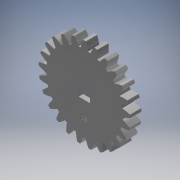
# Autodesk Inventor part: 25_teeth
Saved by Autodesk Inventor 2019 (Build 230136000, 136)
## iProperties
Created: 2020-02-24
Part Number: 25_teeth
Material: Steel
Document SubType Name: Modeling
Designer: Jeff
Categories: <?xml version="1.0" encoding="UTF-16"?> <MemberInstance><Categories><FamilyTemplate><FamilyTemplateParameter ValueType="xs:double" Id="1" ObjectReferenceKey="da_z" ObjectType="kUserParameterObject"/><FamilyTemplateParameter ValueType="xs:double" Id="2" ObjectReferenceKey="da_b" ObjectType="kUserParameterObject"/><FamilyTemplateParameter ValueType="xs:double" Id="3" ObjectReferenceKey="da_beta" ObjectType="kUserParameterObject"/><FamilyTemplateParameter ValueType="xs:double" Id="4" ObjectReferenceKey="da_da" ObjectType="kUserParameterObject"/><FamilyTemplateParameter ValueType="xs:double" Id="5" ObjectReferenceKey="da_aw" ObjectType="kUserParameterObject"/><FamilyTemplateParameter ValueType="xs:string" Id="6" ObjectReferenceKey="EAIAABAAAACIAQAAAAAAAIAAAAAAAAAA" ObjectType="83910656" SubObjectId="SurfaceGeometry"/></FamilyTemplate><ParamToTemplateMap><ParamToTemplate CategoryParameter="//CategoryParameter[@InternalName='046C89C9-8512-4d59-83FE-43B91F4F132A']" TemplateParameter="1"/><ParamToTemplate CategoryParameter="//CategoryParameter[@InternalName='2552DF32-E462-4b46-AEBF-C6C7768E72AC']" TemplateParameter="2"/><ParamToTemplate CategoryParameter="//CategoryParameter[@InternalName='C9EE641D-15FC-4fae-A226-E94C4372FDD7']" TemplateParameter="3"/><ParamToTemplate><ParamToTemplate CategoryParameter="//CategoryParameter[@InternalName='00B6519A-459B-49c7-AD84-2E56D39A5744']" ConstantValue="0.000000"/></ParamToTemplate><ParamToTemplate><ParamToTemplate CategoryParameter="//CategoryParameter[@InternalName='04B31F0E-C7A6-4894-AA32-9629BEFACF47']" ConstantValue="1.000000"/></ParamToTemplate><ParamToTemplate><ParamToTemplate CategoryParameter="//CategoryParameter[@InternalName='43CBEC2E-7847-49e7-A936-2F7889FCB2D9']" ConstantValue="0.250000"/></ParamToTemplate><ParamToTemplate><ParamToTemplate CategoryParameter="//CategoryParameter[@InternalName='B1EFC894-105D-4ebd-86BF-FA20ED196853']" ConstantValue="0.350000"/></ParamToTemplate><ParamToTemplate><ParamToTemplate CategoryParameter="//CategoryParameter[@InternalName='51175063-3D10-4879-93E8-6246FE8B403D']" ConstantValue="2060000000.000000"/></ParamToTemplate><ParamToTemplate><ParamToTemplate CategoryParameter="//CategoryParameter[@InternalName='A3A52E27-4454-46a9-B0BD-C932399B70AF']" ConstantValue="0.300000"/></ParamToTemplate><ParamToTemplate><ParamToTemplate CategoryParameter="//CategoryParameter[@InternalName='91B76062-C214-41d9-B1B9-14D2AB99603D']" ConstantValue="0.300000"/></ParamToTemplate><ParamToTemplate><ParamToTemplate CategoryParameter="//CategoryParameter[@InternalName='374E806E-8B8A-4dda-A9AA-1039D6500AD2']" ConstantValue="3.333333"/></ParamToTemplate><ParamToTemplate><ParamToTemplate CategoryParameter="//CategoryParameter[@InternalName='2D373A89-B862-43d6-8D0B-0CBF12AB9F6C']" ConstantValue="0.349066"/></ParamToTemplate><ParamToTemplate CategoryParameter="//CategoryParameter[@InternalName='37777632-D6A2-4fac-9D53-DB8ACD95C989']" TemplateParameter="4"/><ParamToTemplate CategoryParameter="//CategoryParameter[@InternalName='FD1017F1-B727-4f7e-9707-0F86F1FF9423']" TemplateParameter="5"/><ParamToTemplate><ParamToTemplate CategoryParameter="//CategoryParameter[@InternalName='9E1B4470-B2D3-4ff1-B813-535BB4CDF51A']" ConstantValue="3520000.000000"/></ParamToTemplate><ParamToTemplate><ParamToTemplate CategoryParameter="//CategoryParameter[@InternalName='F8452263-BFF6-458c-9FB1-07C4B99E95CD']" ConstantValue="11400000.000000"/></ParamToTemplate><ParamToTemplate><ParamToTemplate CategoryParameter="//CategoryParameter[@InternalName='3E3BB259-FD49-497f-8171-6EBC954A3479']" ConstantValue="2.000000"/></ParamToTemplate><ParamToTemplate CategoryParameter="//CategoryParameter[@InternalName='27C3BAF2-7550-4e4b-AE2C-0DB134B7D9B7']" TemplateParameter="6"/></ParamToTemplateMap><Category DisplayName="Gear" InternalName="DC85795E-93AB-48d5-8EEE-5A27447B64BD" Mnemonic="Gear"><CategoryParameter DisplayName="z" InternalName="046C89C9-8512-4d59-83FE-43B91F4F132A" Mnemonic="z"/><CategoryParameter DisplayName="b" InternalName="2552DF32-E462-4b46-AEBF-C6C7768E72AC" Mnemonic="b"/><CategoryParameter DisplayName="||b|" InternalName="C9EE641D-15FC-4fae-A226-E94C4372FDD7" Mnemonic="beta"/><CategoryParameter DisplayName="x" InternalName="00B6519A-459B-49c7-AD84-2E56D39A5744" Mnemonic="x"/><CategoryParameter DisplayName="a*" InternalName="04B31F0E-C7A6-4894-AA32-9629BEFACF47" Mnemonic="a"/><CategoryParameter DisplayName="c*" InternalName="43CBEC2E-7847-49e7-A936-2F7889FCB2D9" Mnemonic="c"/><CategoryParameter DisplayName="r|.f|*" InternalName="B1EFC894-105D-4ebd-86BF-FA20ED196853" Mnemonic="rf"/><CategoryParameter DisplayName="E" InternalName="51175063-3D10-4879-93E8-6246FE8B403D" Mnemonic="E"/><CategoryParameter DisplayName="||m|" InternalName="A3A52E27-4454-46a9-B0BD-C932399B70AF" Mnemonic="mi"/><Category DisplayName="SpurGear" InternalName="26C5A22E-A91E-4dfd-A3B3-23CCAFAE1764" Mnemonic="SpurGear"><CategoryParameter DisplayName="m" InternalName="91B76062-C214-41d9-B1B9-14D2AB99603D" Mnemonic="m"/><CategoryParameter DisplayName="P" InternalName="374E806E-8B8A-4dda-A9AA-1039D6500AD2" Mnemonic="PP"/><CategoryParameter DisplayName="||a|" InternalName="2D373A89-B862-43d6-8D0B-0CBF12AB9F6C" Mnemonic="alpha"/><CategoryParameter DisplayName="d|.a|" InternalName="37777632-D6A2-4fac-9D53-DB8ACD95C989" Mnemonic="da"/><CategoryParameter DisplayName="a|.w|" InternalName="FD1017F1-B727-4f7e-9707-0F86F1FF9423" Mnemonic="aw"/><CategoryParameter DisplayName="||s||.Flim|" InternalName="9E1B4470-B2D3-4ff1-B813-535BB4CDF51A" Mnemonic="sFlim"/><CategoryParameter DisplayName="||s||.Hlim|" InternalName="F8452263-BFF6-458c-9FB1-07C4B99E95CD" Mnemonic="sHlim"/><CategoryParameter DisplayName="type" InternalName="3E3BB259-FD49-497f-8171-6EBC954A3479" Mnemonic="type"/><CategoryParameter DisplayName="PitchDiameter" InternalName="27C3BAF2-7550-4e4b-AE2C-0DB134B7D9B7" Mnemonic="IDS_PITCHDIAM"/></Category></Category></Categories></MemberInstance>
Density: 1 g/cm^3
Appearance: Steel
CustomPartVersion: 1
Author: Jeff
Autodesk Inventor part; units mm, degrees
sketch "Sketch1" plane through (0, 0, 0) normal (0, 0, 1) x (1, 0, 0)
  circle A0 centre (0, 0) radius 40.5
  dimension "d0" = 81
  constraints: 1 centre point
  measures "d0" diameter of A0
extrude "Extrusion1" add sketch "Sketch1" along normal blind 10
ref_plane "Work Plane2" through (0, 0, 5) normal (0, 0, 1) x (1, 0, 0)
sketch "Sketch2" plane through (0, 0, 0) normal (0, 0, -1) x (-1, 0, 0)
  circle A0 centre (0, 0) radius 40.5 projected
  circle A1 centre (0, 0) radius 37.5
  dimension "d3" = 75
  constraints: 1 centre point, 1 coincident
  measures "d3" diameter of A1
surface extrude "Pitch Diameter" sketch "Sketch2" against normal through all shown no curves A1
ref_plane "Work Plane8" through (0, 0, 0) normal (0.9921147, 0.1253332, 0) x (0, 0, 1)
ref_plane "Work Plane9" through (0, 0, 0) normal (1, 0, 0) x (0, 1, 0)
spur gear teeth "Spur Gear" teeth 25 pitch diameter 75 tip diameter 81 root diameter 67.5 face width 10 start plane through (0, 0, 0) normal (0, 0, -1) x (-1, 0, 0)
sketch "Sketch3" plane through (0, 0, 10) normal (0, 0, 1) x (1, 0, 0)
  line L0 (-5, 5) -> (5, 5)
  line L1 (5, 5) -> (5, -5)
  line L2 (5, -5) -> (-5, -5)
  line L3 (-5, -5) -> (-5, 5)
  line L4 (-5, -24.3667) -> (-5, -14.3667) construction
  line L5 (-5, -14.3667) -> (5, -14.3667) construction
  line L6 (5, -14.3667) -> (5, -24.3667) construction
  line L7 (5, -24.3667) -> (-5, -24.3667) construction
  arc A0 (-1.0601, -33.7333) -> (1.0601, -33.7333) centre (0, 0) ccw projected
  line L8 (-1.0601, -33.7333) -> (-1.0601, -5)
  line L9 (-0.1823, -20.8667) -> (-2.0324, -20.8667)
  line L10 (-2.0324, -20.8667) -> (-2.0324, -20.4412)
  spline S0 degree 2 poles (-2.0324, -20.4412) (-1.8331, -20.254) (-1.4781, -19.9064) (-1.3079, -19.7192) knots 0 0 0 1 2 2 2
  spline S1 degree 2 poles (-1.3079, -19.7192) (-0.9652, -19.3424) (-0.7147, -18.8902) (-0.7147, -18.6495) knots 0 0 0 1 2 2 2
  spline S2 degree 2 poles (-0.7147, -18.6495) (-0.7147, -18.5231) (-0.7925, -18.3334) (-0.863, -18.2727) knots 0 0 0 1 2 2 2
  spline S3 degree 2 poles (-0.863, -18.2727) (-0.9335, -18.2119) (-1.1183, -18.1511) (-1.2301, -18.1511) knots 0 0 0 1 2 2 2
  spline S4 degree 2 poles (-1.2301, -18.1511) (-1.3371, -18.1511) (-1.5559, -18.2046) (-1.6556, -18.2459) knots 0 0 0 1 2 2 2
  spline S5 degree 2 poles (-1.6556, -18.2459) (-1.7407, -18.28) (-1.8987, -18.3772) (-1.9473, -18.4112) knots 0 0 0 1 2 2 2
  line L11 (-1.9473, -18.4112) -> (-1.9692, -18.4112)
  line L12 (-1.9692, -18.4112) -> (-1.9692, -17.9834)
  spline S6 degree 2 poles (-1.9692, -17.9834) (-1.8452, -17.9226) (-1.4003, -17.8035) (-1.201, -17.8035) knots 0 0 0 1 2 2 2
  spline S7 degree 2 poles (-1.201, -17.8035) (-0.7804, -17.8035) (-0.3063, -18.2484) (-0.3063, -18.6276) knots 0 0 0 1 2 2 2
  spline S8 degree 2 poles (-0.3063, -18.6276) (-0.3063, -18.8051) (-0.389, -19.1017) (-0.4619, -19.2281) knots 0 0 0 1 2 2 2
  spline S9 degree 2 poles (-0.4619, -19.2281) (-0.5348, -19.3594) (-0.7464, -19.6171) (-0.863, -19.7411) knots 0 0 0 1 2 2 2
  spline S10 degree 2 poles (-0.863, -19.7411) (-1.0527, -19.9477) (-1.517, -20.3902) (-1.6556, -20.519) knots 0 0 0 1 2 2 2
  line L13 (-1.6556, -20.519) -> (-0.1823, -20.519)
  line L14 (-0.1823, -20.519) -> (-0.1823, -20.8667)
  spline S11 degree 2 poles (2.0373, -19.9137) (2.0373, -20.13) (1.8987, -20.4996) (1.7723, -20.6357) knots 0 0 0 1 2 2 2
  spline S12 degree 2 poles (1.7723, -20.6357) (1.6459, -20.7719) (1.269, -20.9299) (1.0357, -20.9299) knots 0 0 0 1 2 2 2
  spline S13 degree 2 poles (1.0357, -20.9299) (0.8217, -20.9299) (0.4036, -20.8351) (0.2504, -20.7597) knots 0 0 0 1 2 2 2
  line L15 (0.2504, -20.7597) -> (0.2504, -20.3343)
  line L16 (0.2504, -20.3343) -> (0.2796, -20.3343)
  spline S14 degree 2 poles (0.2796, -20.3343) (0.3258, -20.3683) (0.4984, -20.4558) (0.6029, -20.4947) knots 0 0 0 1 2 2 2
  spline S15 degree 2 poles (0.6029, -20.4947) (0.722, -20.536) (0.919, -20.5822) (1.0429, -20.5822) knots 0 0 0 1 2 2 2
  spline S16 degree 2 poles (1.0429, -20.5822) (1.1645, -20.5822) (1.393, -20.4947) (1.4757, -20.3999) knots 0 0 0 1 2 2 2
  spline S17 degree 2 poles (1.4757, -20.3999) (1.5511, -20.3099) (1.6288, -20.0717) (1.6288, -19.9112) knots 0 0 0 1 2 2 2
  spline S18 degree 2 poles (1.6288, -19.9112) (1.6288, -19.7508) (1.5413, -19.5466) (1.4587, -19.4785) knots 0 0 0 1 2 2 2
  spline S19 degree 2 poles (1.4587, -19.4785) (1.3736, -19.4031) (1.1207, -19.3399) (0.9676, -19.3399) knots 0 0 0 1 2 2 2
  spline S20 degree 2 poles (0.9676, -19.3399) (0.8023, -19.3399) (0.4741, -19.391) (0.3744, -19.4129) knots 0 0 0 1 2 2 2
  line L17 (0.3744, -19.4129) -> (0.3744, -17.8667)
  line L18 (0.3744, -17.8667) -> (2.0203, -17.8667)
  line L19 (2.0203, -17.8667) -> (2.0203, -18.2192)
  line L20 (2.0203, -18.2192) -> (0.7609, -18.2192)
  line L21 (0.7609, -18.2192) -> (0.7609, -19.019)
  spline S21 degree 2 poles (0.7609, -19.019) (0.8339, -19.0093) (0.9749, -19.002) (1.0332, -19.002) knots 0 0 0 1 2 2 2
  spline S22 degree 2 poles (1.0332, -19.002) (1.2642, -19.002) (1.5827, -19.0774) (1.7285, -19.1892) knots 0 0 0 1 2 2 2
  spline S23 degree 2 poles (1.7285, -19.1892) (1.8768, -19.301) (2.0373, -19.6414) (2.0373, -19.9137) knots 0 0 0 1 2 2 2
  point P0 (0, 5)
  point P1 (5, 0)
  point P2 (0, -14.3667)
  point P3 (-5, -19.3667)
  point P4 (-1.0601, -19.3667)
  dimension "d49" = 10
  dimension "d50" = 10
  dimension "d56" = 10
  dimension "d57" = 10
  constraints: 10 end point, 5 midpoint, 2 horizontal, 2 horizontal alignment, 2 parallel, 2 perpendicular, 1 point on line, 1 vertical alignment, 2 other
  measures "d49" distance of L1.end L2.end
  measures "d50" distance of L0.end L1.end
  measures "d56" distance between parallel lines of L6 L4
  measures "d57" distance between parallel lines of L5 L7
extrude "Extrusion2" cut sketch "Sketch3" against normal blind 4 contours L0 L1 L2 L3 | L9 L10 S0 S1 L8 S10 L13 | L8 L13 L14 L9 | L8 S1 S2 S3 S7 S8 S9 S10 | S3 S4 S5 L11 L12 S6 S7 L8 | S11 S12 S13 L15 L16 S14 S15 S16 S17 S18 S19 S20 L17 L18 L19 L20 L21 S21 S22 S23
sketch "Sketch4" plane through (0, 0, 0) normal (0, 0, -1) x (-1, 0, 0)
  circle A0 centre (0, 0) radius 7.5
  dimension "d53" = 15
  constraints: 1 centre point, 1 coincident
  measures "d53" diameter of A0
extrude "Extrusion3" cut sketch "Sketch4" against normal blind 4
equation "\"d0\" = da_da"
equation "\"d1\" = da_b"
equation "\"d3\" = da_dw"
equation "\"d16\" = da_aw"
equation "\"d43\" = da_aw"
equation "\"d46\" = da_aw"
equation "\"da_da\" = 81"
equation "\"da_b\" = 10"
equation "\"da_dw\" = 75"
equation "\"da_aw\" = 52.5"
body "Solid1"
body "Srf1"
